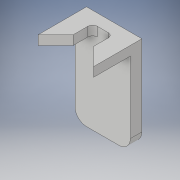
# Autodesk Inventor part: Cable managment.
Saved by Autodesk Inventor 2017 (Build 210142000, 142)
## iProperties
Created: 2018-10-10
Part Number: Cable managment.
Material: Generic
Document SubType Name: Modeling
Designer: Delta
Density: 1 g/cm^3
Appearance: Default
Author: Delta
Autodesk Inventor part; units mm, degrees
ref_plane "YZ Plane" through (0, 0, 0) normal (1, 0, 0) x (0, 1, 0)
ref_plane "XZ Plane" through (0, 0, 0) normal (0, 1, 0) x (-1, 0, 0)
ref_plane "XY Plane" through (0, 0, 0) normal (0, 0, 1) x (1, 0, 0)
sketch "Sketch1" plane through (0, 0, 0) normal (0, 0, 1) x (1, 0, 0)
  line L0 (0, 0) -> (15.24, 0)
  line L1 (15.24, 0) -> (15.24, 25.4)
  line L2 (15.24, 25.4) -> (0, 25.4)
  line L3 (0, 25.4) -> (0, 0)
  dimension "d0" = 15.24
  dimension "d1" = 25.4
  constraints: 8 end point, 2 parallel, 1 horizontal, 1 perpendicular
  measures "d0" distance of L2.end L1.end
  measures "d1" distance of L1.end L0.end
extrude "Extrusion1" add sketch "Sketch1" along normal blind 3.175
sketch "Sketch2" plane through (0, 0, 3.175) normal (0, 0, 1) x (1, 0, 0)
  line L0 (15.24, 25.4) -> (0, 25.4) projected
  line L1 (0, 25.4) -> (4.826, 25.4)
  line L2 (4.826, 25.4) -> (4.826, 22.86)
  line L3 (4.826, 22.86) -> (0, 22.86)
  line L4 (0, 22.86) -> (0, 25.4)
  line L5 (15.24, 25.4) -> (0, 25.4) projected
  line L6 (15.24, 25.4) -> (10.414, 25.4)
  line L7 (10.414, 25.4) -> (10.414, 22.86)
  line L8 (10.414, 22.86) -> (15.24, 22.86)
  line L9 (15.24, 22.86) -> (15.24, 25.4)
  point P0 (0, 0)
  dimension "d4" = 4.826
  dimension "d5" = 2.54
  dimension "d6" = 4.826
  constraints: 16 end point, 4 parallel, 2 horizontal, 2 perpendicular, 1 point on line
  measures "d4" distance of L2.end L3.end
  measures "d5" distance of L1.end L2.end
  measures "d6" distance of L8.end L7.end
extrude "Extrusion2" add sketch "Sketch2" along normal blind 10.16
chamfer "Chamfer1" distance 4.826 angle 45 2 edges at (4.826, 24.13, 13.335) (10.414, 24.13, 13.335)
fillet "Fillet1" radius 1.27 2 edges at (4.826, 24.13, 3.175) (10.414, 24.13, 3.175)
fillet "Fillet2" radius 3.175 2 edges at (15.24, 0, 1.5875) (0, 0, 1.5875)
body "Solid1"
